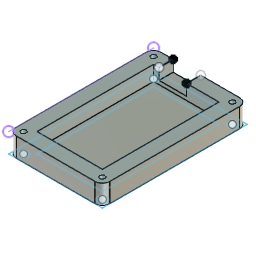
updated macropad v2 (Autodesk Fusion 360 design; units mm, degrees)
Autodesk Fusion 360 part; units mm, degrees
sketch "Sketch1" plane through (0, 0, 0) normal (0, 0, 1) x (1, 0, 0)
  line L0 (-22.3324, 39.6708) -> (21.5296, 39.6708)
  line L1 (21.5296, 39.6708) -> (21.5296, -38.5602)
  line L2 (21.5296, -38.5602) -> (-22.3324, -38.5602)
  line L3 (-22.3324, -38.5602) -> (-22.3324, 39.6708)
  line L4 (-31.8324, 49.1708) -> (31.0296, 49.1708)
  line L5 (31.0296, 49.1708) -> (31.0296, -48.0602)
  line L6 (31.0296, -48.0602) -> (-31.8324, -48.0602)
  line L7 (-31.8324, -48.0602) -> (-31.8324, 49.1708)
  circle A0 centre (-26.8324, 44.1708) radius 1.7
  circle A1 centre (-26.8324, -43.0602) radius 1.7
  circle A2 centre (-26.8324, 44.1708) radius 1.7
  circle A3 centre (26.0296, 44.1708) radius 1.7
  circle A4 centre (26.0296, -43.0602) radius 1.7
  circle A5 centre (26.0296, 44.1708) radius 1.7
  circle A6 centre (-26.8324, 44.1708) radius 3
  circle A7 centre (26.0296, 44.1708) radius 3
  circle A8 centre (26.0296, -43.0602) radius 3
  circle A9 centre (-26.8324, -43.0602) radius 3
  dimension "d1" = 43.862
  dimension "d2" = 78.231
  dimension "d3" = 62.862
  dimension "d4" = 97.231
  dimension "d5" = 9.5
  dimension "d6" = 9.5
  dimension "d7" = 3.4
  dimension "d8" = 5
  dimension "d9" = 5
  dimension "d10" = 3.4
  dimension "d11" = 3.4
  dimension "d12" = 5
  dimension "d13" = 5
  dimension "d14" = 3.4
  dimension "d15" = 5
  dimension "d16" = 5
  dimension "d17" = 3.4
  dimension "d18" = 3.4
  dimension "d19" = 5
  dimension "d20" = 5
  dimension "d21" = 6
  dimension "d22" = 6
  dimension "d23" = 6
  dimension "d24" = 6
  constraint horizontal L0
  constraint vertical L1
  constraint horizontal L2
  constraint vertical L3
  constraint horizontal L4
  constraint vertical L5
  constraint horizontal L6
  constraint vertical L7
  constraint concentric A2 A6
  constraint concentric A3 A7
  constraint concentric A4 A8
  constraint concentric A1 A9
  measures "d1" distance of L0.start L0.end
  measures "d2" distance of L0.start L2.end
  measures "d3" distance of L4.start L4.end
  measures "d4" distance of L4.start L6.end
  measures "d5" distance of L3 L7
  measures "d6" distance of L0 L4
  measures "d7" diameter of A0
  measures "d8" distance of L4 A0.centre
  measures "d9" distance of L7 A0.centre
  measures "d10" diameter of A1
  measures "d11" diameter of A2
  measures "d12" distance of L6 A1.centre
  measures "d13" distance of L7 A1.centre
  measures "d14" diameter of A3
  measures "d15" distance of L4 A3.centre
  measures "d16" distance of L5 A3.centre
  measures "d17" diameter of A4
  measures "d18" diameter of A5
  measures "d19" distance of L5 A4.centre
  measures "d20" distance of L6 A4.centre
  measures "d21" diameter of A6
  measures "d22" diameter of A7
  measures "d23" diameter of A8
  measures "d24" diameter of A9
extrude "Extrude1" add sketch "Sketch1" along normal blind 9.9 from surface at 3.1 contours A6 | A7 | A8 | A9 makes body 1 at (23.0333, 44.0212, 9.7) makes body 2 at (29.0259, -43.2098, 9.7) makes body 3 at (-23.8361, 44.0212, 9.7) makes body 4 at (-23.8361, -43.2098, 9.7)
extrude "Extrude2" add sketch "Sketch1" along normal blind 13 contours L4 L5 L6 L7 bodies 1 2 3 4
extrude "Extrude3" add sketch "Sketch1" along normal blind 3 contours L0 L1 L2 L3 bodies 1
sketch "Sketch2" plane through (0, 0, 13) normal (0, 0, 1) x (-1, 0, 0)
  circle A0 centre (-26.0296, -44.1708) radius 1.7
  circle A1 centre (26.8324, 43.0602) radius 1.7
  line L0 (-21.5296, 38.5602) -> (22.3324, 38.5602)
  line L1 (22.3324, 38.5602) -> (22.3324, -39.6708)
  line L2 (22.3324, -39.6708) -> (-21.5296, -39.6708)
  line L3 (-21.5296, -39.6708) -> (-21.5296, 38.5602)
  line L4 (31.8324, 48.0602) -> (-31.0296, 48.0602)
  line L5 (-31.0296, 48.0602) -> (-31.0296, -49.1708)
  line L6 (-31.0296, -49.1708) -> (31.8324, -49.1708)
  line L7 (31.8324, -49.1708) -> (31.8324, 48.0602)
  circle A2 centre (-26.0296, 43.0602) radius 1.7
  circle A3 centre (26.8324, -44.1708) radius 1.7
  line L8 (0.1714, -49.1708) -> (0.1714, -39.6708)
  line L9 (18.6714, -39.6708) -> (18.6714, -49.1708)
  line L10 (31.8324, 48.0602) -> (31.8324, -49.1708)
  dimension "d32" = 18.5
  dimension "d33" = 13.161
  constraint vertical L8
  constraint vertical L9
  constraint coincident L2 L8.end
  constraint coincident L6 L9.end
  measures "d32" distance of L8 L9
  measures "d33" distance of L9 L10
extrude "Extrude4" cut sketch "Sketch2" against normal blind 7.5 contours L2 L6 L8 L9 bodies 1
fillet "Fillet1" radius 5 1 edges at (-31.8324, 49.1708, 6.5) on bodies 1
fillet "Fillet2" radius 5 1 edges at (31.0296, -48.0602, 6.5) on bodies 1
fillet "Fillet3" radius 5 1 edges at (31.0296, 49.1708, 6.5) on bodies 1
fillet "Fillet4" radius 5 1 edges at (-31.8324, -48.0602, 6.5) on bodies 1
sketch "Sketch3" plane through (0, 0, 13) normal (0, 0, 1) x (-1, 0, 0)
  circle A0 centre (26.8324, -44.1708) radius 1.7
  circle A1 centre (-26.0296, 43.0602) radius 1.7
  arc A2 (31.8324, 43.0602) -> (26.8324, 48.0602) centre (26.8324, 43.0602) ccw
  line L0 (26.8324, 48.0602) -> (-26.0296, 48.0602)
  arc A3 (-26.0296, 48.0602) -> (-31.0296, 43.0602) centre (-26.0296, 43.0602) ccw
  line L1 (-31.0296, 43.0602) -> (-31.0296, -44.1708)
  arc A4 (-31.0296, -44.1708) -> (-26.0296, -49.1708) centre (-26.0296, -44.1708) ccw
  line L2 (-26.0296, -49.1708) -> (0.1714, -49.1708)
  line L3 (0.1714, -49.1708) -> (0.1714, -39.6708)
  line L4 (0.1714, -39.6708) -> (-21.5296, -39.6708)
  line L5 (-21.5296, -39.6708) -> (-21.5296, 38.5602)
  line L6 (-21.5296, 38.5602) -> (22.3324, 38.5602)
  line L7 (22.3324, 38.5602) -> (22.3324, -39.6708)
  line L8 (22.3324, -39.6708) -> (18.6714, -39.6708)
  line L9 (18.6714, -39.6708) -> (18.6714, -49.1708)
  line L10 (18.6714, -49.1708) -> (26.8324, -49.1708)
  arc A5 (26.8324, -49.1708) -> (31.8324, -44.1708) centre (26.8324, -44.1708) ccw
  line L11 (31.8324, -44.1708) -> (31.8324, 43.0602)
  circle A6 centre (26.8324, 43.0602) radius 1.7
  circle A7 centre (-26.0296, -44.1708) radius 1.7
sketch "Sketch4" plane through (0, 0, 0) normal (0, 0, 1) x (1, 0, 0)
  line L0 (-17, -42) -> (12, -42) construction
  line L1 (12, -42) -> (12, -45) construction
  line L2 (12, -45) -> (-17, -45) construction
  line L3 (-17, -45) -> (-17, -42) construction
  dimension "d44" = 2
  text T0 "Vedansh Mannem" font "Arial" height 2 align left top in box 29 x 3 at (-17, -42) x (1, 0) y (0, -1) spacing 1 kerned
extrude "Extrude5" cut sketch "Sketch4" along normal blind 0.2 text T0 bodies 1
equation "d45 = 'Vedansh Mannem'"
